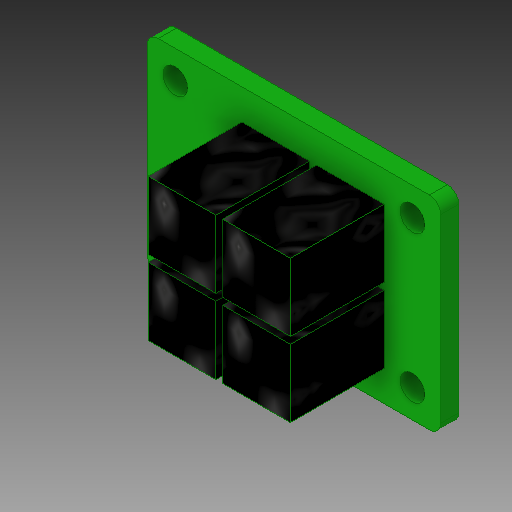
# Autodesk Inventor part: 中継ハブ
Saved by Autodesk Inventor 2017 (Build 210142000, 142)
## iProperties
Created: 2016-08-19
Part Number: 中継ハブ
Material: GFRC
Document SubType Name: Modeling
Designer: NN
Density: 1.7 g/cm^3
Appearance: 濃い緑
Mass: 3.25256 g
Surface Area: 18.9678 cm^2
Volume: 1.91327 cm^3
Author: NN
Autodesk Inventor part; units mm, degrees
ref_plane "YZ Plane" through (0, 0, 0) normal (1, 0, 0) x (0, 1, 0)
ref_plane "XZ Plane" through (0, 0, 0) normal (0, 1, 0) x (-1, 0, 0)
ref_plane "XY Plane" through (0, 0, 0) normal (0, 0, 1) x (1, 0, 0)
sketch "スケッチ1" plane through (0, 0, 0) normal (0, 0, 1) x (1, 0, 0)
  line L0 (0, 0) -> (26, 0)
  line L1 (26, 0) -> (26, 18)
  line L2 (26, 18) -> (0, 18)
  line L3 (0, 18) -> (0, 0)
  dimension "d0" = 26
  dimension "d1" = 18
  constraints: 8 end point, 2 parallel, 1 horizontal, 1 perpendicular
  measures "d0" distance of L0.start L0.end
  measures "d1" distance of L2.end L0.start
extrude "押し出し1" add sketch "スケッチ1" along normal blind 1.6
sketch "スケッチ2" plane through (0, 0, 1.6) normal (0, 0, 1) x (1, 0, 0)
  line L0 (0, 0) -> (26, 0) projected
  line L1 (26, 0) -> (26, 18) projected
  line L2 (26, 18) -> (0, 18) projected
  line L3 (0, 18) -> (0, 0) projected
  line L4 (23.5, 2.5) -> (2.5, 2.5)
  line L5 (2.5, 2.5) -> (2.5, 15.5)
  line L6 (2.5, 15.5) -> (23.5, 15.5)
  line L7 (23.5, 15.5) -> (23.5, 2.5)
  dimension "d4" = 2.5
  constraints: 8 end point, 3 other
  measures "d4" distance between parallel lines of L0 L4
hole "穴1" at (23.5, 15.5, 1.6) at (23.5, 2.5, 1.6) at (2.5, 2.5, 1.6) at (2.5, 15.5, 1.6) direction (0, 0, -1) diameter 2.2 end through all
fillet "フィレット1" radius 1 4 edges at (0, 0, 0.8) (26, 0, 0.8) (0, 18, 0.8) (26, 18, 0.8)
sketch "スケッチ4" plane through (0, 0, 1.6) normal (0, 0, 1) x (1, 0, 0)
  circle A0 centre (2.5, 2.5) radius 1.1 projected
  circle A1 centre (23.5, 15.5) radius 1.1 projected
  circle A2 centre (23.5, 2.5) radius 1.1 projected
  circle A3 centre (2.5, 15.5) radius 1.1 projected
  arc A4 (26, 17) -> (25, 18) centre (25, 17) ccw projected
  line L0 (25, 18) -> (1, 18) projected
  arc A5 (1, 18) -> (0, 17) centre (1, 17) ccw projected
  line L1 (0, 17) -> (0, 1) projected
  arc A6 (0, 1) -> (1, 0) centre (1, 1) ccw projected
  line L2 (1, 0) -> (25, 0) projected
  arc A7 (25, 0) -> (26, 1) centre (25, 1) ccw projected
  line L3 (26, 1) -> (26, 17) projected
  line L4 (15, 15.3) -> (21, 15.3)
  line L5 (21, 15.3) -> (21, 9.3)
  line L6 (21, 9.3) -> (15, 9.3)
  line L7 (15, 9.3) -> (15, 15.3)
  line L8 (26, 1) -> (26, 17) projected
  line L9 (26, 9) -> (14.7, 9)
  line L10 (15, 2.7) -> (21, 2.7)
  line L11 (21, 2.7) -> (21, 8.7)
  line L12 (21, 8.7) -> (15, 8.7)
  line L13 (15, 8.7) -> (15, 2.7)
  line L14 (14.7, 9) -> (14.7, 10.3555)
  line L15 (14.4, 15.3) -> (8.4, 15.3)
  line L16 (8.4, 15.3) -> (8.4, 9.3)
  line L17 (8.4, 9.3) -> (14.4, 9.3)
  line L18 (14.4, 9.3) -> (14.4, 15.3)
  line L19 (14.4, 8.7) -> (14.4, 2.7)
  line L20 (14.4, 2.7) -> (8.4, 2.7)
  line L21 (8.4, 8.7) -> (14.4, 8.7)
  line L22 (8.4, 2.7) -> (8.4, 8.7)
  point P0 (0, 0)
  dimension "d24" = 6
  dimension "d25" = 6
  dimension "d26" = 0.6
  dimension "d27" = 0.6
  dimension "d28" = 5
  constraints: 36 end point, 12 symmetric about line, 2 horizontal, 2 parallel, 1 midpoint, 1 perpendicular, 1 vertical
  measures "d24" distance of L4.start L4.end
  measures "d25" distance of L4.end L5.end
  measures "d26" distance between parallel lines of L6 L12
  measures "d27" distance between parallel lines of L7 L18
  measures "d28" distance between parallel lines of L3 L5
extrude "押し出し2" add sketch "スケッチ4" along normal blind 8.3 contours L4 L5 L6 L7 | L13 L12 L11 L10 | L18 L17 L16 L15 | L19 L20 L22 L21
sketch "スケッチ6" plane through (0, 0, 1.6) normal (0, 0, 1) x (1, 0, 0)
  line L0 (0, 17) -> (0, 1) projected
  line L1 (0, 9) -> (6.7, 9)
  line L2 (6.7, 9) -> (6.7, 11.5)
  circle A0 centre (6.7, 11.5) radius 0.8483
  circle A1 centre (6.7, 9) radius 0.8884
  circle A2 centre (6.7, 6.5) radius 0.8483
  circle A3 centre (6.7, 9) radius 0.8884
  point P0 (0, 0)
  dimension "d33" = 6.7
  dimension "d34" = 2.5
  dimension "d35" = 0
  constraints: 4 centre point, 4 end point, 2 symmetric about line, 1 coincident, 1 horizontal, 1 midpoint, 1 perpendicular, 1 point on line, 2 other
  measures "d33" distance between parallel lines of L0 L2
  measures "d34" distance of A1.centre L2.end
  measures "d35" distance of A3.centre A1.centre
hole "穴3" at (6.7, 11.5, 1.6) at (6.7, 9, 1.6) at (6.7, 9, 1.6) at (6.7, 6.5, 1.6) direction (0, 0, -1) diameter 1 end through all
sketch "スケッチ8" plane through (0, 0, 1.6) normal (0, 0, 1) x (1, 0, 0)
  circle A0 centre (6.7, 9) radius 0.5 projected
  circle A1 centre (6.7, 11.5) radius 0.5 projected
  circle A2 centre (6.7, 6.5) radius 0.5 projected
  line L0 (14.4, 15.3) -> (14.4, 9.3) projected
  line L1 (14.4, 9.3) -> (8.4, 9.3) projected
  line L2 (8.4, 9.3) -> (8.4, 15.3) projected
  line L3 (8.4, 15.3) -> (14.4, 15.3) projected
  line L4 (21, 15.3) -> (21, 9.3) projected
  line L5 (21, 9.3) -> (15, 9.3) projected
  line L6 (15, 9.3) -> (15, 15.3) projected
  line L7 (15, 15.3) -> (21, 15.3) projected
  line L8 (21, 8.7) -> (21, 2.7) projected
  line L9 (21, 2.7) -> (15, 2.7) projected
  line L10 (15, 2.7) -> (15, 8.7) projected
  line L11 (15, 8.7) -> (21, 8.7) projected
  line L12 (14.4, 8.7) -> (14.4, 2.7) projected
  line L13 (14.4, 2.7) -> (8.4, 2.7) projected
  line L14 (8.4, 2.7) -> (8.4, 8.7) projected
  line L15 (8.4, 8.7) -> (14.4, 8.7) projected
  circle A3 centre (2.5, 2.5) radius 1.1 projected
  circle A4 centre (23.5, 15.5) radius 1.1 projected
  circle A5 centre (23.5, 2.5) radius 1.1 projected
  circle A6 centre (2.5, 15.5) radius 1.1 projected
  arc A7 (26, 17) -> (25, 18) centre (25, 17) ccw projected
  line L16 (25, 18) -> (1, 18) projected
  arc A8 (1, 18) -> (0, 17) centre (1, 17) ccw projected
  line L17 (0, 17) -> (0, 1) projected
  arc A9 (0, 1) -> (1, 0) centre (1, 1) ccw projected
  line L18 (1, 0) -> (25, 0) projected
  arc A10 (25, 0) -> (26, 1) centre (25, 1) ccw projected
  line L19 (26, 1) -> (26, 17) projected
  line L20 (6.7, 6.5) -> (6.7, 4)
  circle A11 centre (6.7, 4) radius 0.5842
  point P0 (0, 0)
  dimension "d44" = 2.5
  constraints: 2 end point, 1 centre point, 1 coincident, 1 vertical
  measures "d44" distance of L20.start L20.end
hole "穴4" at (6.7, 4, 1.6) direction (0, 0, -1) diameter 1 end through all
